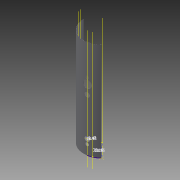
# Autodesk Inventor part: EDM Middle Shield Part 2
Saved by Autodesk Inventor 2015 (Build 190159000, 159)
## iProperties
Created: 2014-06-18
Part Number: EDM Middle Shield Part 2
Material: Generic
Document SubType Name: Modeling
Designer: Aki
Density: 1 g/cm^3
Appearance: Default
Author: Aki
Autodesk Inventor part; units mm, degrees
ref_plane "YZ Plane" through (0, 0, 0) normal (1, 0, 0) x (0, 1, 0)
sketch "Sketch1" plane through (0, 0, 0) normal (0, 1, 0) x (-1, 0, 0)
  arc A0 (307.3366, -1.4483) -> (-211.0135, 223.4528) centre (0, 0) ccw
  line L0 (0, 0) -> (-211.0135, 223.4528) construction
  line L1 (0, 0) -> (307.3366, -1.4483) construction
  arc A1 (306.0666, -1.4423) -> (-210.1416, 222.5295) centre (0, 0) ccw
  line L2 (0, 0) -> (306.0666, -1.4423) construction
  line L3 (0, 0) -> (-210.1416, 222.5295) construction
  line L4 (-210.1416, 222.5295) -> (-211.0135, 223.4528)
  line L5 (307.3366, -1.4483) -> (306.0666, -1.4423)
  dimension "d0" = 307.34
  dimension "d1" = 133.63
  dimension "d2" = 306.07
  dimension "d3" = 133.63
  constraints: 12 end point, 4 point on circle, 2 centre point, 2 coincident, 1 collinear, 1 point on line
  measures "d0" radius of A0
  measures "d1" angle of L1 L0
  measures "d2" radius of A1
  measures "d3" angle of L2 L3
extrude "Extrusion1" add sketch "Sketch1" along normal blind 1625.6
sketch "Sketch2" plane through (0, 0, 0) normal (0, 1, 0) x (-1, 0, 0)
  arc A0 (307.3366, -1.4483) -> (303.3865, 49.1379) centre (0, 0) ccw
  line L0 (0, 0) -> (303.3865, 49.1379) construction
  line L1 (0, 0) -> (307.3366, -1.4483) construction
  dimension "d6" = 9.47
  constraints: 4 end point, 2 point on circle, 1 centre point, 1 coincident
  measures "d6" angle of L1 L0
ref_plane "Work Plane1" through (-303.3865, 0, 49.1379) normal (-0.9871363, 0, 0.1598812) x (0, -1, 0)
sketch "Sketch3" plane through (-303.3865, 0, 49.1379) normal (-0.9871363, 0, 0.1598812) x (0, -1, 0)
  circle A0 centre (-158.75, 0) radius 88.9
  line L0 (0, 307.34) -> (0, -50.567) projected
  line L1 (-247.65, 0) -> (-69.85, 0)
  line L2 (-69.85, 0) -> (-69.85, -88.9)
  line L3 (-69.85, -88.9) -> (-247.65, -88.9)
  line L4 (-247.65, -88.9) -> (-247.65, 0)
  point P0 (0, 0)
  point P1 (0, 254.3155)
  dimension "d7" = 177.8
  dimension "d8" = 158.75
  constraints: 8 end point, 2 parallel, 1 horizontal, 1 horizontal alignment, 1 perpendicular, 2 other
  measures "d8" distance from line of L0 point (-158.75, 0)
extrude "Extrusion2" cut sketch "Sketch3" against normal blind 25.4
sketch "Sketch4" plane through (0, 0, 0) normal (0, 1, 0) x (-1, 0, 0)
  arc A0 (-54.4252, 302.4827) -> (-211.0135, 223.4528) centre (0, 0) ccw
  line L0 (0, 0) -> (-54.4252, 302.4827) construction
  line L1 (0, 0) -> (-211.0135, 223.4528) construction
  dimension "d11" = 33.16
  constraints: 4 end point, 2 point on circle, 1 centre point, 1 coincident
  measures "d11" angle of L0 L1
ref_plane "Work Plane2" through (54.4252, 0, 302.4827) normal (0.1770847, 0, 0.9841956) x (0, 1, 0)
sketch "Sketch5" plane through (54.4252, 0, 302.4827) normal (0.1770847, 0, 0.9841956) x (0, 1, 0)
  circle A0 centre (158.75, 0) radius 25.4
  line L0 (0, -168.1085) -> (0, 307.34) projected
  circle A1 centre (234.95, 0) radius 38.1
  circle A2 centre (871.5375, 0) radius 38.1
  circle A3 centre (1022.35, 0) radius 63.5
  circle A4 centre (1120.775, 0) radius 25.4
  point P0 (0, 0)
  point P1 (0, 302.2228)
  dimension "d12" = 50.8
  dimension "d13" = 158.75
  dimension "d14" = 76.2
  dimension "d15" = 234.95
  dimension "d16" = 76.2
  dimension "d17" = 871.5375
  dimension "d18" = 127
  dimension "d19" = 1022.35
  dimension "d20" = 50.8
  dimension "d21" = 1120.775
  constraints: 5 centre point
  measures "d12" diameter of A0
  measures "d13" distance from line of L0 A0.centre
  measures "d14" diameter of A1
  measures "d15" distance of point (0, 0) A1.centre
  measures "d16" diameter of A2
  measures "d17" distance from line of L0 A2.centre
  measures "d18" diameter of A3
  measures "d19" distance from line of L0 A3.centre
  measures "d20" diameter of A4
  measures "d21" distance from line of L0 A4.centre
extrude "Extrusion3" cut sketch "Sketch5" against normal blind 25.4
sketch "Sketch6" plane through (0, 0, 0) normal (0, 1, 0) x (-1, 0, 0)
  arc A0 (-127.0124, 279.8674) -> (-211.0135, 223.4528) centre (0, 0) ccw
  line L0 (0, 0) -> (-127.0124, 279.8674) construction
  line L1 (0, 0) -> (-211.0135, 223.4528) construction
  arc A1 (307.34, 0) -> (290.6829, 99.8065) centre (0, 0) ccw
  line L2 (0, 0) -> (290.6829, 99.8065) construction
  line L3 (0, 0) -> (307.34, 0) construction
  dimension "d24" = 18.95
  dimension "d25" = 18.95
  constraints: 8 end point, 4 point on circle, 2 centre point, 2 coincident
  measures "d24" angle of L0 L1
  measures "d25" angle of L3 L2
body "Solid1"
